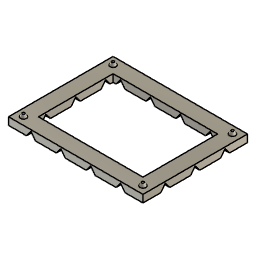
Grooved v3 (Autodesk Fusion 360 design; units mm, degrees)
Autodesk Fusion 360 part; units mm, degrees
sketch "Sketch1" plane through (0, 0, 0) normal (0, 0, 1) x (1, 0, 0)
  line L0 (-45, 35) -> (45, 35)
  line L1 (45, 35) -> (45, -35)
  line L2 (45, -35) -> (-45, -35)
  line L3 (-45, -35) -> (-45, 35)
  line L4 (-45, 35) -> (45, -35) construction
  line L5 (45, 35) -> (-45, -35) construction
  line L6 (-35, 25) -> (35, 25)
  line L7 (35, 25) -> (35, -25)
  line L8 (35, -25) -> (-35, -25)
  line L9 (-35, -25) -> (-35, 25)
  line L10 (-35, 25) -> (35, -25) construction
  line L11 (35, 25) -> (-35, -25) construction
  dimension "d1" = 90
  dimension "d2" = 70
  dimension "d3" = 10
  dimension "d4" = 10
  constraint horizontal L0
  constraint perpendicular L0 L1
  constraint parallel L0 L2
  constraint parallel L1 L3
  constraint coincident L4 origin
  constraint coincident L5 origin
  constraint horizontal L6
  constraint perpendicular L6 L7
  constraint parallel L6 L8
  constraint parallel L7 L9
  constraint coincident L10 origin
  constraint coincident L11 origin
  measures "d1" distance of L0.start L0.end
  measures "d2" distance of L0.start L2.end
  measures "d3" distance of L3 L9
  measures "d4" distance of L0 L6
extrude "Extrude1" add sketch "Sketch1" along normal blind 5
sketch "Sketch2" plane through (0, -35, 0) normal (0, -1, 0) x (1, 0, 0)
  line L0 (-45, 0) -> (45, 0)
  line L1 (45, 0) -> (45, 5)
  line L2 (45, 5) -> (-45, 5)
  line L3 (-33, 0) -> (-30, 4)
  line L4 (-30, 4) -> (-27, 0)
  line L5 (-33, 0) -> (-27, 0)
  dimension "d37" = 4
  dimension "d40" = 15
  dimension "d41" = 6
  constraint coincident L0 L3.start
  constraint coincident L0 L4.end
  constraint equal L3 L4
  constraint coincident L3.end L4.start
  measures "d37" vertical distance of L3.start L3.end
  measures "d40" horizontal distance of L2.end L3.end
  measures "d41" distance of L3.start L4.end
extrude "Extrude2" cut sketch "Sketch2" against normal through all
pattern_linear "R-Pattern1" count 4 spacing 20 along (1, 0, 0) of "Extrude2"
sketch "Sketch3" plane through (-45, 0, 0) normal (-1, 0, 0) x (0, -1, 0)
  line L0 (-35, 0) -> (35, 0)
  line L1 (35, 0) -> (35, 5)
  line L2 (35, 5) -> (-35, 5)
  line L3 (-23, 0) -> (-20, 4)
  line L4 (-20, 4) -> (-17, 0)
  dimension "d42" = 6
  dimension "d43" = 4
  dimension "d44" = 15
  constraint coincident L0 L3.start
  constraint coincident L0 L4.end
  constraint equal L3 L4
  measures "d42" distance of L3.start L4.end
  measures "d43" distance of L0 L3.end
  measures "d44" horizontal distance of L2.end L3.end
extrude "Extrude3" cut sketch "Sketch3" against normal through all
pattern_linear "R-Pattern2" count 3 spacing 20 along (0, -1, 0) of "Extrude3"
sketch "Sketch4" plane through (0, 0, 5) normal (0, 0, 1) x (-1, 0, 0)
  line L0 (45, -35) -> (45, 35)
  line L1 (45, 35) -> (-45, 35)
  line L2 (-35, 25) -> (35, 25)
  line L3 (35, 25) -> (35, -25)
  circle A0 centre (40, 30) radius 2
  line L4 (35, -25) -> (-35, -25)
  line L5 (-35, -25) -> (-35, 25)
  line L6 (-45, 35) -> (-45, -35)
  line L7 (-45, -35) -> (45, -35)
  dimension "d23" = 5
  dimension "d24" = 5
  dimension "d25" = 4
  measures "d23" distance of L0 A0.centre
  measures "d24" distance of L1 A0.centre
  measures "d25" diameter of A0
extrude "Extrude4" add sketch "Sketch4" along normal blind 2 draft -30 contours A0
sketch "Sketch5" plane through (0, 0, 0) normal (0, 0, -1) x (1, 0, 0)
  circle A0 centre (-40, 30) radius 2
  line L0 (45, -23) -> (35, -23)
  line L1 (-45, 35) -> (-45, 23)
  line L2 (33, -35) -> (45, -35)
  line L3 (-33, 25) -> (-33, 35)
  line L4 (35, -25) -> (33, -25)
  line L5 (-35, 23) -> (-35, 25)
  line L6 (35, -23) -> (35, -25)
  line L7 (33, -25) -> (33, -35)
  line L8 (45, -35) -> (45, -23)
  line L9 (-33, 35) -> (-45, 35)
  line L10 (-45, 35) -> (-45, 23)
  line L11 (-45, 23) -> (-35, 23)
  line L12 (-35, 25) -> (-33, 25)
  line L13 (-33, 35) -> (-45, 35)
  line L14 (35, 23) -> (45, 23)
  line L15 (45, 23) -> (45, 35)
  line L16 (45, 35) -> (33, 35)
  line L17 (33, 35) -> (33, 25)
  line L18 (33, 25) -> (35, 25)
  line L19 (35, 25) -> (35, 23)
  line L20 (-35, -23) -> (-45, -23)
  line L21 (-45, -23) -> (-45, -35)
  line L22 (-45, -35) -> (-33, -35)
  line L23 (-33, -35) -> (-33, -25)
  line L24 (-33, -25) -> (-35, -25)
  line L25 (-35, -25) -> (-35, -23)
  dimension "d30" = 4
  dimension "d45" = 5
  dimension "d46" = 5
  measures "d30" diameter of A0
  measures "d45" distance of A0.centre L9
  measures "d46" distance of A0.centre L10
extrude "Extrude5" cut sketch "Sketch5" against normal blind 2 draft -30 contours A0
pattern_linear "R-Pattern3" count 2 spacing 80 along (1, 0, 0) count 2 spacing 60 along (0, 1, 0) of "Extrude4", "Extrude5"
